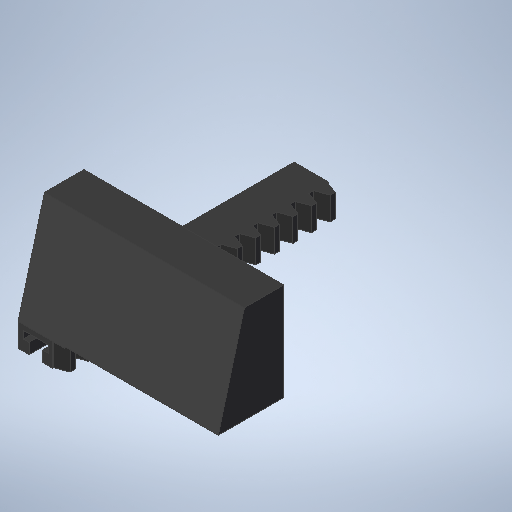
# Autodesk Inventor part: sg90 claw v2 finger
Saved by Autodesk Inventor 2025 (Build 290162000, 162)
## iProperties
Created: 2025-05-11
Part Number: sg90 claw v2 finger
Material: 一般
Document SubType Name: Modeling
Designer: gavin
Density: 1 g/cm^3
Appearance: 預設
Author: gavin
## iProperties of the stored document sg90 claw v2 finger_3D 列印.ipt
Created: 2025-05-11
Part Number: sg90 claw v2 finger_3D 列印
Material: 一般
Document SubType Name: Modeling
Designer: gavin
Density: 1 g/cm^3
Appearance: 預設
Author: gavin
Autodesk Inventor part; units mm, degrees
ref_plane "YZ Plane" through (0, 0, 0) normal (1, 0, 0) x (0, 1, 0)
ref_plane "XZ Plane" through (0, 0, 0) normal (0, 1, 0) x (-1, 0, 0)
sketch "草圖1" plane through (0, 0, 0) normal (0, 0, 1) x (1, 0, 0)
  line L0 (0, -4.2926) -> (-50, -4.2926) projected
  line L1 (0, -4.2926) -> (0, 3.81) projected
  line L2 (0, 3.81) -> (-2.5, 3.81) projected
  line L3 (-2.5, 3.81) -> (-2.5, 6.9129) projected
  line L4 (-2.5, 6.9129) -> (-1, 6.9129) projected
  line L5 (-1, 6.9129) -> (-1, 8.4129) projected
  line L6 (-1, 8.4129) -> (-7, 8.4129) projected
  line L7 (-7, 8.4129) -> (-7, 6.9129) projected
  line L8 (-7, 6.9129) -> (-5.5, 6.9129) projected
  line L9 (-5.5, 6.9129) -> (-5.5, 3.81) projected
  line L10 (-5.5, 3.81) -> (-44.5, 3.81) projected
  line L11 (-44.5, 3.81) -> (-44.5, 6.9129) projected
  line L12 (-44.5, 6.9129) -> (-43, 6.9129) projected
  line L13 (-43, 6.9129) -> (-43, 8.4129) projected
  line L14 (-43, 8.4129) -> (-49, 8.4129) projected
  line L15 (-49, 8.4129) -> (-49, 6.9129) projected
  line L16 (-49, 6.9129) -> (-47.5, 6.9129) projected
  line L17 (-47.5, 6.9129) -> (-47.5, 3.81) projected
  line L18 (-47.5, 3.81) -> (-50, 3.81) projected
  line L19 (-50, -4.2926) -> (-50, 3.81) projected
  line L20 (-44.3, 6.7129) -> (-44.3, 4.01)
  line L21 (-44.3, 4.01) -> (-5.7, 4.01)
  line L22 (-5.7, 4.01) -> (-5.7, 6.7129)
  line L23 (-5.7, 6.7129) -> (-7.2, 6.7129)
  line L24 (-7.2, 6.7129) -> (-7.2, 8.6129)
  line L25 (-7.2, 8.6129) -> (-0.8, 8.6129)
  line L26 (-0.8, 8.6129) -> (-0.8, 6.7129)
  line L27 (-0.8, 6.7129) -> (-2.3, 6.7129)
  line L28 (-2.3, 6.7129) -> (-2.3, 4.01)
  line L29 (-2.3, 4.01) -> (0.2, 4.01)
  line L30 (0.2, 4.01) -> (0.2, -4.4926)
  line L31 (0.2, -4.4926) -> (-50.2, -4.4926)
  line L32 (-50.2, -4.4926) -> (-50.2, 4.01)
  line L33 (-50.2, 4.01) -> (-47.7, 4.01)
  line L34 (-47.7, 4.01) -> (-47.7, 6.7129)
  line L35 (-47.7, 6.7129) -> (-49.2, 6.7129)
  line L36 (-49.2, 6.7129) -> (-49.2, 8.6129)
  line L37 (-49.2, 8.6129) -> (-42.8, 8.6129)
  line L38 (-42.8, 8.6129) -> (-42.8, 6.7129)
  line L39 (-42.8, 6.7129) -> (-44.3, 6.7129)
  line L40 (-50.2, 4.01) -> (-50.2, 9.9129)
  line L41 (-50.2, 9.9129) -> (-41.8, 9.9129)
  line L42 (-41.8, 9.9129) -> (-41.8, 4.01)
  line L43 (-41.8, 6.7405) -> (-41.8, 4.0405)
  point P0 (0, 0)
  point P1 (-41.8, 5.3905)
  dimension "d0" = 0.2
  dimension "d3" = 1
  dimension "d4" = 1.3
  constraints: 48 end point, 2 perpendicular, 2 point on line, 1 midpoint, 1 vertical, 19 other
  measures "d0" distance between parallel lines of L11 L20
  measures "d3" distance between parallel lines of L42 L38
  measures "d4" distance between parallel lines of L37 L41
ref_plane "工作平面1" through (-50, -4.2926, -70) normal (0, 0, -1) x (0, 1, 0)
extrude "擠出1" add sketch "草圖1" against normal up to surface (70 mm away) contours L39 L38 L37 L36 L35 L34 L33 L40 L41 L42 L21 L20
sketch "草圖2" plane through (-50.2, 9.9129, 0) normal (0, 1, 0) x (1, 0, 0)
  line L0 (8.4617, 19.101) -> (11.5117, 20.2111)
  line L1 (11.5117, 20.2111) -> (11.5117, 21.4754)
  line L2 (11.5117, 21.4754) -> (8.4617, 22.5855)
  line L3 (8.4617, 22.5855) -> (8.4617, 23.8134)
  line L4 (8.4617, 23.8134) -> (11.5117, 24.9235)
  line L5 (11.5117, 24.9235) -> (11.5117, 26.1878)
  line L6 (11.5117, 26.1878) -> (8.4617, 27.2979)
  line L7 (8.4617, 27.2979) -> (8.4617, 28.5258)
  line L8 (8.4617, 28.5258) -> (11.5117, 29.6359)
  line L9 (11.5117, 29.6359) -> (11.5117, 30.9002)
  line L10 (11.5117, 30.9002) -> (8.4617, 32.0103)
  line L11 (8.4617, 32.0103) -> (8.4617, 33.2382)
  line L12 (8.4617, 33.2382) -> (11.5117, 34.3483)
  line L13 (11.5117, 34.3483) -> (11.5117, 35.6126)
  line L14 (11.5117, 35.6126) -> (8.4617, 36.7227)
  line L15 (8.4617, 36.7227) -> (8.4617, 37.9506)
  line L16 (8.4617, 37.9506) -> (11.5117, 39.0607)
  line L17 (11.5117, 39.0607) -> (11.5117, 40.325)
  line L18 (11.5117, 40.325) -> (8.4617, 41.4351)
  line L19 (8.4617, 41.4351) -> (8.4617, 42.663)
  line L20 (8.4617, 42.663) -> (11.5117, 43.7731)
  line L21 (11.5117, 43.7731) -> (11.5117, 45.0373)
  line L22 (11.5117, 45.0373) -> (8.4617, 46.1475)
  line L23 (8.4617, 46.1475) -> (8.4617, 47.3753)
  line L24 (8.4617, 47.3753) -> (11.5117, 48.4855)
  line L25 (11.5117, 48.4855) -> (11.5117, 49.7497)
  line L26 (11.5117, 49.7497) -> (8.4617, 50.8598)
  circle A0 centre (25.2, 35) radius 1.15 projected
  spline S0 degree 3 poles (28.303, 18.8298) (28.3918, 19.076) (28.7004, 19.9315) (28.7388, 21.2949) (28.6496, 21.419) (28.6524, 21.7961) (28.6611, 21.9313) (28.7622, 22.2015) (28.8309, 22.282) (28.9256, 22.387) (29.0049, 22.4333) (29.139, 22.5114) (29.2816, 22.5522) (29.5147, 22.6052) (29.6038, 22.5977) (29.679, 22.5914) (29.7699, 22.5777) (29.9387, 22.4894) (30.0374, 22.4306) (30.278, 22.1628) (30.3615, 21.9889) (30.5339, 21.6254) (30.761, 21.3363) (31.4807, 20.5784) (31.9907, 20.2322) (32.1942, 20.0941) knots 0 0 0 0 0.078525 0.078525 0.123346 0.123346 0.136441 0.136441 0.149096 0.149096 0.177084 0.177084 0.558526 0.558526 0.807734 0.807734 2.330173 2.330173 3.026337 3.026337 3.902772 3.902772 11.004243 11.004243 24.626338 24.626338 24.626338 24.626338 projected
  arc A1 (32.1942, 20.0941) -> (33.148, 20.5801) centre (25.2, 35) ccw projected
  spline S1 degree 3 poles (33.148, 20.5801) (33.1564, 20.8417) (33.1855, 21.7507) (32.8007, 23.0592) (32.6775, 23.1497) (32.5637, 23.5092) (32.5301, 23.6405) (32.5428, 23.9287) (32.5833, 24.0265) (32.6409, 24.1556) (32.702, 24.2241) (32.8054, 24.3399) (32.9285, 24.4227) (33.1337, 24.5452) (33.2208, 24.5656) (33.2942, 24.5828) (33.3849, 24.5979) (33.5727, 24.566) (33.6848, 24.5406) (33.9964, 24.3602) (34.1295, 24.2207) (34.4058, 23.9282) (34.7112, 23.7235) (35.6298, 23.2251) (36.2218, 23.0535) (36.458, 22.985) knots 0 0 0 0 0.078525 0.078525 0.123346 0.123346 0.136441 0.136441 0.149096 0.149096 0.177084 0.177084 0.558526 0.558526 0.807734 0.807734 2.330173 2.330173 3.026337 3.026337 3.902772 3.902772 11.004243 11.004243 24.626338 24.626338 24.626338 24.626338 projected
  arc A2 (36.458, 22.985) -> (37.215, 23.742) centre (25.2, 35) ccw projected
  spline S2 degree 3 poles (37.215, 23.742) (37.1421, 23.9934) (36.889, 24.8668) (36.1186, 25.9924) (35.9735, 26.0404) (35.7541, 26.3471) (35.6817, 26.4616) (35.6047, 26.7396) (35.6129, 26.8451) (35.6278, 26.9857) (35.6648, 27.0698) (35.7273, 27.2118) (35.8188, 27.3286) (35.9762, 27.5085) (36.0526, 27.5549) (36.1172, 27.5939) (36.1988, 27.6363) (36.3872, 27.664) (36.5016, 27.6744) (36.8537, 27.5992) (37.0234, 27.5077) (37.3766, 27.3148) (37.7303, 27.2145) (38.758, 27.0244) (39.3741, 27.0441) (39.6199, 27.052) knots 0 0 0 0 0.078525 0.078525 0.123346 0.123346 0.136441 0.136441 0.149096 0.149096 0.177084 0.177084 0.558526 0.558526 0.807734 0.807734 2.330173 2.330173 3.026337 3.026337 3.902772 3.902772 11.004243 11.004243 24.626338 24.626338 24.626338 24.626338 projected
  arc A3 (39.6199, 27.052) -> (40.1059, 28.0058) centre (25.2, 35) ccw projected
  spline S3 degree 3 poles (40.1059, 28.0058) (39.9589, 28.2224) (39.4482, 28.9749) (38.3677, 29.8073) (38.2149, 29.8081) (37.9115, 30.032) (37.8072, 30.1185) (37.648, 30.3591) (37.6233, 30.462) (37.594, 30.6003) (37.6032, 30.6917) (37.6187, 30.8461) (37.6696, 30.9855) (37.7637, 31.2052) (37.8221, 31.2729) (37.8714, 31.33) (37.9359, 31.3955) (38.1066, 31.4801) (38.2122, 31.5254) (38.5703, 31.5626) (38.76, 31.528) (39.1555, 31.4538) (39.5228, 31.4677) (40.559, 31.6044) (41.1388, 31.8135) (41.3702, 31.897) knots 0 0 0 0 0.078525 0.078525 0.123346 0.123346 0.136441 0.136441 0.149096 0.149096 0.177084 0.177084 0.558526 0.558526 0.807734 0.807734 2.330173 2.330173 3.026337 3.026337 3.902772 3.902772 11.004243 11.004243 24.626338 24.626338 24.626338 24.626338 projected
  arc A4 (41.3702, 31.897) -> (41.5376, 32.9543) centre (25.2, 35) ccw projected
  spline S4 degree 3 poles (41.5376, 32.9543) (41.3309, 33.1148) (40.6127, 33.6727) (39.3279, 34.1305) (39.1823, 34.0841) (38.8245, 34.2032) (38.6986, 34.2532) (38.4729, 34.4329) (38.4176, 34.5231) (38.3469, 34.6456) (38.3275, 34.7353) (38.2946, 34.887) (38.2999, 35.0353) (38.3215, 35.2733) (38.3561, 35.3558) (38.3854, 35.4253) (38.4264, 35.5076) (38.5627, 35.6407) (38.6491, 35.7164) (38.9781, 35.8625) (39.1693, 35.8882) (39.5683, 35.9398) (39.9134, 36.0665) (40.8566, 36.5168) (41.3434, 36.8949) (41.5376, 37.0457) knots 0 0 0 0 0.078525 0.078525 0.123346 0.123346 0.136441 0.136441 0.149096 0.149096 0.177084 0.177084 0.558526 0.558526 0.807734 0.807734 2.330173 2.330173 3.026337 3.026337 3.902772 3.902772 11.004243 11.004243 24.626338 24.626338 24.626338 24.626338 projected
  arc A5 (41.5376, 37.0457) -> (41.3702, 38.103) centre (25.2, 35) ccw projected
  spline S5 degree 3 poles (41.3702, 38.103) (41.124, 38.1918) (40.2685, 38.5004) (38.9051, 38.5388) (38.781, 38.4496) (38.4039, 38.4524) (38.2687, 38.4611) (37.9985, 38.5622) (37.918, 38.6309) (37.813, 38.7256) (37.7667, 38.8049) (37.6886, 38.939) (37.6478, 39.0816) (37.5948, 39.3147) (37.6023, 39.4038) (37.6086, 39.479) (37.6223, 39.5699) (37.7106, 39.7387) (37.7694, 39.8374) (38.0372, 40.078) (38.2111, 40.1615) (38.5746, 40.3339) (38.8637, 40.561) (39.6216, 41.2807) (39.9678, 41.7907) (40.1059, 41.9942) knots 0 0 0 0 0.078525 0.078525 0.123346 0.123346 0.136441 0.136441 0.149096 0.149096 0.177084 0.177084 0.558526 0.558526 0.807734 0.807734 2.330173 2.330173 3.026337 3.026337 3.902772 3.902772 11.004243 11.004243 24.626338 24.626338 24.626338 24.626338 projected
  arc A6 (40.1059, 41.9942) -> (39.6199, 42.948) centre (25.2, 35) ccw projected
  spline S6 degree 3 poles (39.6199, 42.948) (39.3583, 42.9564) (38.4493, 42.9855) (37.1408, 42.6007) (37.0503, 42.4775) (36.6908, 42.3637) (36.5595, 42.3301) (36.2713, 42.3428) (36.1735, 42.3833) (36.0444, 42.4409) (35.9759, 42.502) (35.8601, 42.6054) (35.7773, 42.7285) (35.6548, 42.9337) (35.6344, 43.0208) (35.6172, 43.0942) (35.6021, 43.1849) (35.634, 43.3727) (35.6594, 43.4848) (35.8398, 43.7964) (35.9793, 43.9295) (36.2718, 44.2058) (36.4765, 44.5112) (36.9749, 45.4298) (37.1465, 46.0218) (37.215, 46.258) knots 0 0 0 0 0.078525 0.078525 0.123346 0.123346 0.136441 0.136441 0.149096 0.149096 0.177084 0.177084 0.558526 0.558526 0.807734 0.807734 2.330173 2.330173 3.026337 3.026337 3.902772 3.902772 11.004243 11.004243 24.626338 24.626338 24.626338 24.626338 projected
  arc A7 (37.215, 46.258) -> (36.458, 47.015) centre (25.2, 35) ccw projected
  spline S7 degree 3 poles (36.458, 47.015) (36.2066, 46.9421) (35.3332, 46.689) (34.2076, 45.9186) (34.1596, 45.7735) (33.8529, 45.5541) (33.7384, 45.4817) (33.4604, 45.4047) (33.3549, 45.4129) (33.2143, 45.4278) (33.1302, 45.4648) (32.9882, 45.5273) (32.8714, 45.6188) (32.6915, 45.7762) (32.6451, 45.8526) (32.6061, 45.9172) (32.5637, 45.9988) (32.536, 46.1872) (32.5256, 46.3016) (32.6008, 46.6537) (32.6923, 46.8234) (32.8852, 47.1766) (32.9855, 47.5303) (33.1756, 48.558) (33.1559, 49.1741) (33.148, 49.4199) knots 0 0 0 0 0.078525 0.078525 0.123346 0.123346 0.136441 0.136441 0.149096 0.149096 0.177084 0.177084 0.558526 0.558526 0.807734 0.807734 2.330173 2.330173 3.026337 3.026337 3.902772 3.902772 11.004242 11.004242 24.626338 24.626338 24.626338 24.626338 projected
  arc A8 (33.148, 49.4199) -> (32.1942, 49.9059) centre (25.2, 35) ccw projected
  spline S8 degree 3 poles (32.1942, 49.9059) (31.9776, 49.7589) (31.2251, 49.2482) (30.3927, 48.1677) (30.3919, 48.0149) (30.168, 47.7115) (30.0815, 47.6072) (29.8409, 47.448) (29.738, 47.4233) (29.5997, 47.394) (29.5083, 47.4032) (29.3539, 47.4187) (29.2145, 47.4696) (28.9948, 47.5637) (28.9271, 47.6221) (28.87, 47.6714) (28.8045, 47.7359) (28.7199, 47.9066) (28.6746, 48.0122) (28.6374, 48.3703) (28.672, 48.56) (28.7462, 48.9555) (28.7323, 49.3228) (28.5956, 50.359) (28.3865, 50.9388) (28.303, 51.1702) knots 0 0 0 0 0.078525 0.078525 0.123346 0.123346 0.136441 0.136441 0.149096 0.149096 0.177084 0.177084 0.558526 0.558526 0.807734 0.807734 2.330173 2.330173 3.026337 3.026337 3.902772 3.902772 11.004243 11.004243 24.626338 24.626338 24.626338 24.626338 projected
  arc A9 (28.303, 51.1702) -> (27.2457, 51.3376) centre (25.2, 35) ccw projected
  spline S9 degree 3 poles (27.2457, 51.3376) (27.0852, 51.1309) (26.5273, 50.4127) (26.0695, 49.1279) (26.1159, 48.9823) (25.9968, 48.6245) (25.9468, 48.4986) (25.7671, 48.2729) (25.6769, 48.2176) (25.5544, 48.1469) (25.4647, 48.1275) (25.313, 48.0946) (25.1647, 48.0999) (24.9267, 48.1215) (24.8442, 48.1561) (24.7747, 48.1854) (24.6924, 48.2264) (24.5593, 48.3627) (24.4836, 48.4491) (24.3375, 48.7781) (24.3118, 48.9693) (24.2602, 49.3683) (24.1335, 49.7134) (23.6832, 50.6566) (23.3051, 51.1434) (23.1543, 51.3376) knots 0 0 0 0 0.078525 0.078525 0.123346 0.123346 0.136441 0.136441 0.149096 0.149096 0.177084 0.177084 0.558526 0.558526 0.807734 0.807734 2.330173 2.330173 3.026337 3.026337 3.902772 3.902772 11.004243 11.004243 24.626338 24.626338 24.626338 24.626338 projected
  arc A10 (23.1543, 51.3376) -> (22.097, 51.1702) centre (25.2, 35) ccw projected
  spline S10 degree 3 poles (22.097, 51.1702) (22.0082, 50.924) (21.6996, 50.0685) (21.6612, 48.7051) (21.7504, 48.581) (21.7476, 48.2039) (21.7389, 48.0687) (21.6378, 47.7985) (21.5691, 47.718) (21.4744, 47.613) (21.3951, 47.5667) (21.261, 47.4886) (21.1184, 47.4478) (20.8853, 47.3948) (20.7962, 47.4023) (20.721, 47.4086) (20.6301, 47.4223) (20.4613, 47.5106) (20.3626, 47.5694) (20.122, 47.8372) (20.0385, 48.0111) (19.8661, 48.3746) (19.639, 48.6637) (18.9193, 49.4216) (18.4093, 49.7678) (18.2058, 49.9059) knots 0 0 0 0 0.078525 0.078525 0.123346 0.123346 0.136441 0.136441 0.149096 0.149096 0.177084 0.177084 0.558526 0.558526 0.807734 0.807734 2.330173 2.330173 3.026337 3.026337 3.902772 3.902772 11.004242 11.004242 24.626338 24.626338 24.626338 24.626338 projected
  arc A11 (18.2058, 49.9059) -> (17.252, 49.4199) centre (25.2, 35) ccw projected
  spline S11 degree 3 poles (17.252, 49.4199) (17.2436, 49.1583) (17.2145, 48.2493) (17.5993, 46.9408) (17.7225, 46.8503) (17.8363, 46.4908) (17.8699, 46.3595) (17.8572, 46.0713) (17.8167, 45.9735) (17.7591, 45.8444) (17.698, 45.7759) (17.5946, 45.6601) (17.4715, 45.5773) (17.2663, 45.4548) (17.1792, 45.4344) (17.1058, 45.4172) (17.0151, 45.4021) (16.8273, 45.434) (16.7152, 45.4594) (16.4036, 45.6398) (16.2705, 45.7793) (15.9942, 46.0718) (15.6888, 46.2765) (14.7702, 46.7749) (14.1782, 46.9465) (13.942, 47.015) knots 0 0 0 0 0.078525 0.078525 0.123346 0.123346 0.136441 0.136441 0.149096 0.149096 0.177084 0.177084 0.558526 0.558526 0.807734 0.807734 2.330173 2.330173 3.026337 3.026337 3.902772 3.902772 11.004243 11.004243 24.626338 24.626338 24.626338 24.626338 projected
  arc A12 (13.942, 47.015) -> (13.185, 46.258) centre (25.2, 35) ccw projected
  spline S12 degree 3 poles (13.185, 46.258) (13.2579, 46.0066) (13.511, 45.1332) (14.2814, 44.0076) (14.4265, 43.9596) (14.6459, 43.6529) (14.7183, 43.5384) (14.7953, 43.2604) (14.7871, 43.1549) (14.7722, 43.0143) (14.7352, 42.9302) (14.6727, 42.7882) (14.5812, 42.6714) (14.4238, 42.4915) (14.3474, 42.4451) (14.2828, 42.4061) (14.2012, 42.3637) (14.0128, 42.336) (13.8984, 42.3256) (13.5463, 42.4008) (13.3766, 42.4923) (13.0234, 42.6852) (12.6697, 42.7855) (11.642, 42.9756) (11.0259, 42.9559) (10.7801, 42.948) knots 0 0 0 0 0.078525 0.078525 0.123346 0.123346 0.136441 0.136441 0.149096 0.149096 0.177084 0.177084 0.558526 0.558526 0.807734 0.807734 2.330173 2.330173 3.026337 3.026337 3.902772 3.902772 11.004242 11.004242 24.626338 24.626338 24.626338 24.626338 projected
  arc A13 (10.7801, 42.948) -> (10.2941, 41.9942) centre (25.2, 35) ccw projected
  spline S13 degree 3 poles (10.2941, 41.9942) (10.4411, 41.7776) (10.9518, 41.0251) (12.0323, 40.1927) (12.1851, 40.1919) (12.4885, 39.968) (12.5928, 39.8815) (12.752, 39.6409) (12.7767, 39.538) (12.806, 39.3997) (12.7968, 39.3083) (12.7813, 39.1539) (12.7304, 39.0145) (12.6363, 38.7948) (12.5779, 38.7271) (12.5286, 38.67) (12.4641, 38.6045) (12.2934, 38.5199) (12.1878, 38.4746) (11.8297, 38.4374) (11.64, 38.472) (11.2445, 38.5462) (10.8772, 38.5323) (9.841, 38.3956) (9.2612, 38.1865) (9.0298, 38.103) knots 0 0 0 0 0.078525 0.078525 0.123346 0.123346 0.136441 0.136441 0.149096 0.149096 0.177084 0.177084 0.558526 0.558526 0.807734 0.807734 2.330173 2.330173 3.026337 3.026337 3.902772 3.902772 11.004243 11.004243 24.626338 24.626338 24.626338 24.626338 projected
  arc A14 (9.0298, 38.103) -> (8.8624, 37.0457) centre (25.2, 35) ccw projected
  spline S14 degree 3 poles (8.8624, 37.0457) (9.0691, 36.8852) (9.7873, 36.3273) (11.0721, 35.8695) (11.2177, 35.9159) (11.5755, 35.7968) (11.7014, 35.7468) (11.9271, 35.5671) (11.9824, 35.4769) (12.0531, 35.3544) (12.0725, 35.2647) (12.1054, 35.113) (12.1001, 34.9647) (12.0785, 34.7267) (12.0439, 34.6442) (12.0146, 34.5747) (11.9736, 34.4924) (11.8373, 34.3593) (11.7509, 34.2836) (11.4219, 34.1375) (11.2307, 34.1118) (10.8317, 34.0602) (10.4866, 33.9335) (9.5434, 33.4832) (9.0566, 33.1051) (8.8624, 32.9543) knots 0 0 0 0 0.078525 0.078525 0.123346 0.123346 0.136441 0.136441 0.149096 0.149096 0.177084 0.177084 0.558526 0.558526 0.807734 0.807734 2.330173 2.330173 3.026337 3.026337 3.902772 3.902772 11.004243 11.004243 24.626338 24.626338 24.626338 24.626338 projected
  arc A15 (8.8624, 32.9543) -> (9.0298, 31.897) centre (25.2, 35) ccw projected
  spline S15 degree 3 poles (9.0298, 31.897) (9.276, 31.8082) (10.1315, 31.4996) (11.4949, 31.4612) (11.619, 31.5504) (11.9961, 31.5476) (12.1313, 31.5389) (12.4015, 31.4378) (12.482, 31.3691) (12.587, 31.2744) (12.6333, 31.1951) (12.7114, 31.061) (12.7522, 30.9184) (12.8052, 30.6853) (12.7977, 30.5962) (12.7914, 30.521) (12.7777, 30.4301) (12.6894, 30.2613) (12.6306, 30.1626) (12.3628, 29.922) (12.1889, 29.8385) (11.8254, 29.6661) (11.5363, 29.439) (10.7784, 28.7193) (10.4322, 28.2093) (10.2941, 28.0058) knots 0 0 0 0 0.078525 0.078525 0.123346 0.123346 0.136441 0.136441 0.149096 0.149096 0.177084 0.177084 0.558526 0.558526 0.807734 0.807734 2.330173 2.330173 3.026337 3.026337 3.902772 3.902772 11.004243 11.004243 24.626338 24.626338 24.626338 24.626338 projected
  arc A16 (10.2941, 28.0058) -> (10.7801, 27.052) centre (25.2, 35) ccw projected
  spline S16 degree 3 poles (10.7801, 27.052) (11.0417, 27.0436) (11.9507, 27.0145) (13.2592, 27.3993) (13.3497, 27.5225) (13.7092, 27.6363) (13.8405, 27.6699) (14.1287, 27.6572) (14.2265, 27.6167) (14.3556, 27.5591) (14.4241, 27.498) (14.5399, 27.3946) (14.6227, 27.2715) (14.7452, 27.0663) (14.7656, 26.9792) (14.7828, 26.9058) (14.7979, 26.8151) (14.766, 26.6273) (14.7406, 26.5152) (14.5602, 26.2036) (14.4207, 26.0705) (14.1282, 25.7942) (13.9235, 25.4888) (13.4251, 24.5702) (13.2535, 23.9782) (13.185, 23.742) knots 0 0 0 0 0.078525 0.078525 0.123346 0.123346 0.136441 0.136441 0.149096 0.149096 0.177084 0.177084 0.558526 0.558526 0.807734 0.807734 2.330173 2.330173 3.026337 3.026337 3.902772 3.902772 11.004243 11.004243 24.626338 24.626338 24.626338 24.626338 projected
  arc A17 (13.185, 23.742) -> (13.942, 22.985) centre (25.2, 35) ccw projected
  spline S17 degree 3 poles (13.942, 22.985) (14.1934, 23.0579) (15.0668, 23.311) (16.1924, 24.0814) (16.2404, 24.2265) (16.5471, 24.4459) (16.6616, 24.5183) (16.9396, 24.5953) (17.0451, 24.5871) (17.1857, 24.5722) (17.2698, 24.5352) (17.4118, 24.4727) (17.5286, 24.3812) (17.7085, 24.2238) (17.7549, 24.1474) (17.7939, 24.0828) (17.8363, 24.0012) (17.864, 23.8128) (17.8744, 23.6984) (17.7992, 23.3463) (17.7077, 23.1766) (17.5148, 22.8234) (17.4145, 22.4697) (17.2244, 21.442) (17.2441, 20.8259) (17.252, 20.5801) knots 0 0 0 0 0.078525 0.078525 0.123346 0.123346 0.136441 0.136441 0.149096 0.149096 0.177084 0.177084 0.558526 0.558526 0.807734 0.807734 2.330173 2.330173 3.026337 3.026337 3.902772 3.902772 11.004243 11.004243 24.626338 24.626338 24.626338 24.626338 projected
  arc A18 (17.252, 20.5801) -> (18.2058, 20.0941) centre (25.2, 35) ccw projected
  spline S18 degree 3 poles (18.2058, 20.0941) (18.4224, 20.2411) (19.1749, 20.7518) (20.0073, 21.8323) (20.0081, 21.9851) (20.232, 22.2885) (20.3185, 22.3928) (20.5591, 22.552) (20.662, 22.5767) (20.8003, 22.606) (20.8917, 22.5968) (21.0461, 22.5813) (21.1855, 22.5304) (21.4052, 22.4363) (21.4729, 22.3779) (21.53, 22.3286) (21.5955, 22.2641) (21.6801, 22.0934) (21.7254, 21.9878) (21.7626, 21.6297) (21.728, 21.44) (21.6538, 21.0445) (21.6677, 20.6772) (21.8044, 19.641) (22.0135, 19.0612) (22.097, 18.8298) knots 0 0 0 0 0.078525 0.078525 0.123346 0.123346 0.136441 0.136441 0.149096 0.149096 0.177084 0.177084 0.558526 0.558526 0.807734 0.807734 2.330173 2.330173 3.026337 3.026337 3.902772 3.902772 11.004243 11.004243 24.626338 24.626338 24.626338 24.626338 projected
  arc A19 (22.097, 18.8298) -> (23.1543, 18.6624) centre (25.2, 35) ccw projected
  spline S19 degree 3 poles (23.1543, 18.6624) (23.3148, 18.8691) (23.8727, 19.5873) (24.3305, 20.8721) (24.2841, 21.0177) (24.4032, 21.3755) (24.4532, 21.5014) (24.6329, 21.7271) (24.7231, 21.7824) (24.8456, 21.8531) (24.9353, 21.8725) (25.087, 21.9054) (25.2353, 21.9001) (25.4733, 21.8785) (25.5558, 21.8439) (25.6253, 21.8146) (25.7076, 21.7736) (25.8407, 21.6373) (25.9164, 21.5509) (26.0625, 21.2219) (26.0882, 21.0307) (26.1398, 20.6317) (26.2665, 20.2866) (26.7168, 19.3434) (27.0949, 18.8566) (27.2457, 18.6624) knots 0 0 0 0 0.078525 0.078525 0.123346 0.123346 0.136441 0.136441 0.149096 0.149096 0.177084 0.177084 0.558526 0.558526 0.807734 0.807734 2.330173 2.330173 3.026337 3.026337 3.902772 3.902772 11.004243 11.004243 24.626338 24.626338 24.626338 24.626338 projected
  arc A20 (27.2457, 18.6624) -> (28.303, 18.8298) centre (25.2, 35) ccw projected
  line L27 (8.4, 70) -> (0, 70) projected
  line L28 (0, 0) -> (0, 70) projected
  line L29 (8.4, 0) -> (0, 0) projected
  line L30 (8.4, 0) -> (8.4, 70) projected
  line L31 (8.4617, 50.8598) -> (8.4617, 52.0877)
  line L32 (8.4617, 52.0877) -> (11.5117, 53.1978)
  line L33 (11.5117, 53.1978) -> (11.5117, 54.4621)
  line L34 (11.5117, 54.4621) -> (8.4617, 55.5722)
  line L35 (8.4617, 55.5722) -> (8.4617, 56.8001)
  line L36 (8.4617, 56.8001) -> (11.5117, 57.9102)
  line L37 (11.5117, 57.9102) -> (11.5117, 59.1745)
  line L38 (11.5117, 59.1745) -> (8.4617, 60.2846)
  line L39 (8.4617, 60.2846) -> (8.4617, 61.5125)
  line L40 (8.4617, 61.5125) -> (11.5117, 62.6226)
  line L41 (11.5117, 62.6226) -> (11.5117, 63.8869)
  line L42 (11.5117, 63.8869) -> (8.4617, 64.997)
  line L43 (8.4617, 64.997) -> (8.4617, 66.2249)
  line L44 (8.4617, 66.2249) -> (11.5117, 67.335)
  line L45 (11.5117, 67.335) -> (11.5117, 68.5993)
  line L46 (11.5117, 68.5993) -> (8.4617, 69.7094)
  line L47 (8.4617, 69.7094) -> (8.4617, 70)
  line L48 (8.4617, 70) -> (8.3127, 70)
  line L49 (8.1638, 0) -> (8.3127, 70)
  line L50 (8.4617, 14.3886) -> (11.5117, 15.4988)
  line L51 (11.5117, 15.4988) -> (11.5117, 16.763)
  line L52 (11.5117, 16.763) -> (8.4617, 17.8731)
  line L53 (8.4617, 17.8731) -> (8.4617, 19.101)
  line L54 (8.4617, 9.6763) -> (11.5117, 10.7864)
  line L55 (11.5117, 10.7864) -> (11.5117, 12.0506)
  line L56 (11.5117, 12.0506) -> (8.4617, 13.1608)
  line L57 (8.4617, 13.1608) -> (8.4617, 14.3886)
  line L58 (8.4617, 4.9639) -> (11.5117, 6.074)
  line L59 (11.5117, 6.074) -> (11.5117, 7.3383)
  line L60 (11.5117, 7.3383) -> (8.4617, 8.4484)
  line L61 (8.4617, 8.4484) -> (8.4617, 9.6763)
  line L62 (8.4617, 0.2515) -> (11.5117, 1.3616)
  line L63 (11.5117, 1.3616) -> (11.5117, 2.6259)
  line L64 (11.5117, 2.6259) -> (8.4617, 3.736)
  line L65 (8.4617, 3.736) -> (8.4617, 4.9639)
  line L66 (8.4617, 0.2515) -> (8.4617, 0)
  line L67 (8.4617, 0) -> (8.1638, 0)
  point P0 (50.2, 0)
  point P1 (8.4617, 3.736)
  point P2 (8.4617, 4.9639)
  point P3 (8.4617, 8.4484)
  point P4 (8.4617, 9.6763)
  point P5 (8.4617, 13.1608)
  point P6 (8.4617, 14.3886)
  point P7 (8.4617, 17.8731)
  point P8 (8.4617, 19.101)
  point P9 (8.4617, 22.5855)
  point P10 (8.4617, 23.8134)
  point P11 (8.4617, 27.2979)
  point P12 (8.4617, 28.5258)
  point P13 (8.4617, 32.0103)
  point P14 (8.4617, 33.2382)
  point P15 (8.4617, 36.7227)
  point P16 (8.4617, 37.9506)
  point P17 (8.4617, 41.4351)
  point P18 (8.4617, 42.663)
  point P19 (8.4617, 46.1475)
  point P20 (8.4617, 47.3753)
  point P21 (8.4617, 50.8598)
  point P22 (8.4617, 52.0877)
  point P23 (8.4617, 55.5722)
  point P24 (8.4617, 56.8001)
  point P25 (8.4617, 60.2846)
  point P26 (8.4617, 61.5125)
  point P27 (8.4617, 64.997)
  point P28 (8.4617, 66.2249)
  constraints: 128 end point, 2 point on line, 1 perpendicular, 1 vertical
extrude "擠出2" add sketch "草圖2" against normal up to surface (5.9029 mm away) contours L53 L52 L51 L50 L57 L56 L55 L54 L61 L60 L59 L58 L65 L64 L63 L62 L66 L67 L30 L48 L47 L46 L45 L44 L43 L42 L41 L40 L39 L38 L37 L36 L35 L34 L33 L32 L31 L26 L25 L24 L23 L22 L21 L20 L19 L18 L17 L16 L15 L14 L13 L12 L11 L10 L9 L8 L7 L6 L5 L4 L3 L2 L1 L0
sketch "草圖3" plane through (-50.2, 4.01, 0) normal (-1, 0, 0) x (0, 0, 1)
  line L0 (0, 5.9029) -> (-70, 5.9029) projected
  line L1 (0, 5.9029) -> (0, 0) projected
  line L2 (0, 5.9029) -> (-6.6987, 30.9029)
  line L3 (-6.6987, 30.9029) -> (-16.6987, 30.9029)
  line L4 (-16.6987, 30.9029) -> (-16.6987, 5.9029)
  point P0 (0, -4.01)
  dimension "d14" = 75
  dimension "d15" = 10
  dimension "d16" = 25
  constraints: 6 end point, 2 perpendicular, 1 point on line
  measures "d14" angle of L0 L2
  measures "d15" distance of L2.end L3.end
  measures "d16" distance of L3.end L4.end
extrude "擠出3" add sketch "草圖3" against normal blind 50.4
sketch "草圖4" plane through (-50.2, 9.9129, -16.6987) normal (0, 0, -1) x (-1, 0, 0)
  line L0 (0, 25) -> (0, 0) projected
  line L1 (0, 25) -> (-50.4, 25) projected
  line L2 (-50.4, 0) -> (-50.4, 25) projected
  line L3 (-11.5117, 0) -> (-50.4, 0) projected
  line L4 (0, 0) -> (-11.5117, 0) projected
  line L5 (-50.4, 0.3) -> (-11.5117, 0.3)
  line L6 (-11.5117, 0.3) -> (-11.5117, 0)
  point P0 (-50.2, -9.9129)
  dimension "d19" = 0.3
  constraints: 4 end point, 1 horizontal, 1 perpendicular, 1 point on line
  measures "d19" distance between parallel lines of L3 L5
extrude "擠出4" cut sketch "草圖4" against normal blind 50.4 contours L3 L2 L5 L6
sketch "草圖5" plane through (-50.2, 4.01, -70) normal (-1, 0, 0) x (0, 0, 1)
  line L0 (0, 5.9029) -> (0, 0) projected
  line L1 (70, 0) -> (0, 0) projected
  line L2 (70, 5.9029) -> (70, 0) projected
  line L3 (70, 5.9029) -> (63.3013, 30.9029) projected
  line L4 (63.3013, 30.9029) -> (53.3013, 30.9029) projected
  line L5 (53.3013, 30.9029) -> (53.3013, 5.9029) projected
  line L6 (53.3013, 5.9029) -> (0, 5.9029) projected
  point P0 (70, -4.01)
extrude "擠出5" add sketch "草圖5" along normal blind 0.3
